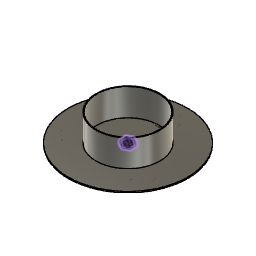
无标题 v6 (Autodesk Fusion 360 design; units mm, degrees)
Autodesk Fusion 360 part; units mm, degrees
sketch "草图1" plane through (0, 0, 0) normal (0, 0, 1) x (1, 0, 0)
  circle A0 centre (0, 0) radius 150
  dimension "d1" = 300
  constraint coincident A0.centre origin
  measures "d1" diameter of A0
extrude "拉伸1" add sketch "草图1" along normal blind 50 makes body 1
sketch "草图2" plane through (0, 0, 50) normal (0, 0, 1) x (-1, 0, 0)
  circle A0 centre (0, 0) radius 150
  circle A1 centre (0, 0) radius 80
  constraint coincident A0.centre A1.centre
extrude "拉伸2" add sketch "草图2" along normal blind 40 contours A1 bodies 1
sketch "草图3" plane through (0, 0, 90) normal (0, 0, 1) x (-1, 0, 0)
  circle A0 centre (0, 0) radius 80
extrude "拉伸3" cut 1 faces at (125.8104, -11.4266, 50) along direction (0, 0, -1) blind 48 on bodies 1 bodies 1
shell "抽壳1" thickness 2 removed faces 1 at (-18.9694, 28.4446, 90) on bodies 1
extrude "拉伸4" add 1 faces at (125.8104, -11.4266, 2) along direction (0, 0, 1) blind 1 on bodies 1 bodies 1
sketch "草图4" plane through (0, 0, 0) normal (0, 1, 0) x (1, 0, 0)
sketch "草图5" plane through (0, 0, 2) normal (0, 0, 1) x (-1, 0, 0)
  circle A0 centre (0, 0) radius 78
sketch "草图6" plane through (0, 0, 2) normal (0, 0, 1) x (1, 0, 0)
  line L0 (13.9361, -0.9993) -> (7.8335, 11.5694)
  line L1 (7.8335, 11.5694) -> (-6.1026, 12.5687)
  line L2 (-6.1026, 12.5687) -> (-13.9361, 0.9993)
  line L3 (-13.9361, 0.9993) -> (-7.8335, -11.5694)
  line L4 (-7.8335, -11.5694) -> (6.1026, -12.5687)
  line L5 (6.1026, -12.5687) -> (13.9361, -0.9993)
  line L6 (-7.6157, 15.6849) -> (-17.3913, 1.2471)
  line L7 (-17.3913, 1.2471) -> (-9.7757, -14.4378)
  line L8 (-9.7757, -14.4378) -> (7.6157, -15.6849)
  line L9 (7.6157, -15.6849) -> (17.3913, -1.2471)
  line L10 (17.3913, -1.2471) -> (9.7757, 14.4378)
  line L11 (9.7757, 14.4378) -> (-7.6157, 15.6849)
  dimension "d37" = 1
  measures "d11" distance of origin L5
sketch "草图7" plane through (0, 0, 2) normal (0, 0, 1) x (-1, 0, 0)
  circle A0 centre (0, 0) radius 78
  line L0 (-6.05, -3.493) -> (0, -6.9859)
  line L1 (0, -6.9859) -> (6.05, -3.493)
  line L2 (6.05, -3.493) -> (6.05, 3.493)
  line L3 (6.05, 3.493) -> (0, 6.9859)
  line L4 (0, 6.9859) -> (-6.05, 3.493)
  line L5 (-6.05, 3.493) -> (-6.05, -3.493)
  line L6 (8.05, 4.6477) -> (0, 9.2953)
  line L7 (0, 9.2953) -> (-8.05, 4.6477)
  line L8 (-8.05, 4.6477) -> (-8.05, -4.6477)
  line L9 (-8.05, -4.6477) -> (0, -9.2953)
  line L10 (0, -9.2953) -> (8.05, -4.6477)
  line L11 (8.05, -4.6477) -> (8.05, 4.6477)
  dimension "d14" = 6.05
  dimension "d15" = 2
  measures "d14" distance of A0.centre L5
sketch "草图8" plane through (0, 0, 2) normal (0, 0, 1) x (-1, 0, 0)
extrude "拉伸5" add sketch "草图7" along normal blind 6 contours L6 L7 L8 L9 L10 L11 bodies 1
sketch "草图9" plane through (0, 0, 0) normal (1, 0, 0) x (0, 1, 0)
extrude "拉伸6" cut 1 faces at (-78.7451, 7.8496, 90) along direction (0, 0, -1) blind 20 on bodies 1 bodies 1
sketch "草图10" plane through (0, 0, 0) normal (0, 0, -1) x (1, 0, 0)
  circle A0 centre (0, 0) radius 150
  line L0 (0, 0) -> (0, -100)
  circle A1 centre (0, -100) radius 26
  circle A2 centre (86.6025, 50) radius 26
  circle A3 centre (-86.6025, 50) radius 26
  dimension "d20" = 100
  dimension "d21" = 52
  dimension "d23" = 360
  constraint coincident A0.centre L0.start
  constraint vertical L0
  constraint coincident L0.end A1.centre
  measures "d20" distance of A0.centre L0.end
  measures "d21" diameter of A1
extrude "拉伸7" cut sketch "草图10" against normal blind 0.01 contours A1 | A2 | A3 bodies 1
sketch "草图11" plane through (0, 0, 0) normal (0, 1, 0) x (1, 0, 0)
extrude "拉伸8" cut 3 faces at (-95.1724, -51.2917, 0.01) (94.3141, -47.5314, 0.01) (-6.5706, 96.6215, 0.01) along direction (0, 0, 1) blind 0.5 on bodies 1 bodies 1
sketch "草图12" plane through (0, 0, 2) normal (0, 0, 1) x (-1, 0, 0)
  circle A0 centre (0, 0) radius 78
  line L0 (8.05, -4.6477) -> (0, -9.2953)
  line L1 (0, -9.2953) -> (-8.05, -4.6477)
  line L2 (-8.05, -4.6477) -> (-8.05, 4.6477)
  line L3 (-8.05, 4.6477) -> (0, 9.2953)
  line L4 (0, 9.2953) -> (8.05, 4.6477)
  line L5 (8.05, 4.6477) -> (8.05, -4.6477)
sketch "草图13" plane through (0, 0, 0) normal (0, 1, 0) x (1, 0, 0)
sketch "草图14" plane through (0, 0, 2) normal (0, 0, 1) x (-1, 0, 0)
extrude "拉伸9" cut 1 faces at (2.6833, -6.9763, 8) along direction (0, 0, -1) blind 7 on bodies 1 bodies 1
sketch "草图15" plane through (0, 0, 2) normal (0, 0, 1) x (-1, 0, 0)
  line L0 (0, -9.2953) -> (-8.05, -4.6477)
  line L1 (8.05, -4.6477) -> (0, -9.2953)
  line L2 (8.05, 4.6477) -> (8.05, -4.6477)
  line L3 (0, 9.2953) -> (8.05, 4.6477)
  line L4 (-8.05, 4.6477) -> (0, 9.2953)
  line L5 (-8.05, -4.6477) -> (-8.05, 4.6477)
  line L6 (-6.05, 3.493) -> (-6.05, -3.493)
  line L7 (-6.05, -3.493) -> (0, -6.9859)
  line L8 (0, -6.9859) -> (6.05, -3.493)
  line L9 (6.05, -3.493) -> (6.05, 3.493)
  line L10 (6.05, 3.493) -> (0, 6.9859)
  line L11 (0, 6.9859) -> (-6.05, 3.493)
  line L12 (6.9515, 4.0134) -> (0, 8.0269)
  line L13 (0, 8.0269) -> (-6.9515, 4.0134)
  line L14 (-6.9515, 4.0134) -> (-6.9515, -4.0134)
  line L15 (-6.9515, -4.0134) -> (0, -8.0269)
  line L16 (0, -8.0269) -> (6.9515, -4.0134)
  line L17 (6.9515, -4.0134) -> (6.9515, 4.0134)
  line L18 (0, -10.5391) -> (-9.1272, -5.2696)
  line L19 (-9.1272, -5.2696) -> (-9.1272, 5.2696)
  line L20 (-9.1272, 5.2696) -> (0, 10.5391)
  line L21 (0, 10.5391) -> (9.1272, 5.2696)
  line L22 (9.1272, 5.2696) -> (9.1272, -5.2696)
  line L23 (9.1272, -5.2696) -> (0, -10.5391)
  circle A0 centre (0, 0) radius 1.55
  dimension "d30" = 0.9015
  dimension "d31" = -1.0772
  dimension "d32" = 3.1
  constraint coincident A0.centre origin
  measures "d32" diameter of A0
extrude "拉伸10" add sketch "草图15" along normal blind 6 contours L0 L1 L2 L3 L4 L5 | L18 L19 L20 L21 L22 L23 bodies 1
sketch "草图16" plane through (0, 0, 2) normal (0, 0, 1) x (-1, 0, 0)
  circle A0 centre (0, 0) radius 2.2585
  constraint coincident A0.centre origin
extrude "拉伸11" cut sketch "草图16" against normal blind 13 bodies 1
chamfer "倒角1" distance 1 angle 45 6 edges at (-6.9515, 0, 8) (-3.4757, 6.0202, 8) (3.4757, 6.0202, 8) (6.9515, 0, 8) (3.4757, -6.0202, 8) (-3.4757, -6.0202, 8) on bodies 1
extrude "拉伸12" add sketch "草图15" along normal blind 0.5 separate body contours L12 L13 L14 L15 L16 L17 makes body 2
